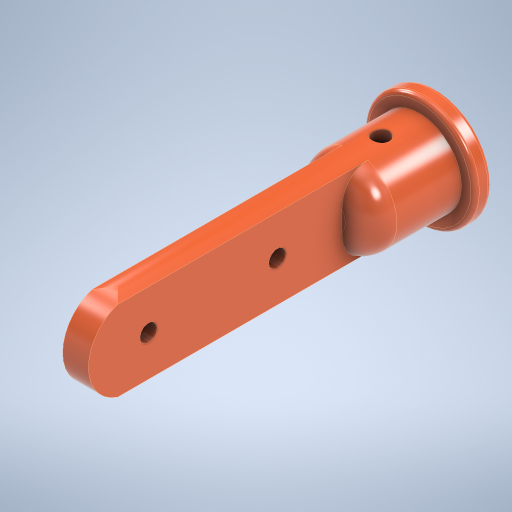
# Autodesk Inventor part: pin
Saved by Autodesk Inventor 2023.2 (Build 272271000, 271)
## iProperties
Created: 2022-11-27
Part Number: pin
Material: Generic
Document SubType Name: Modeling
Designer: omrfrkmll
Density: 1 g/cm^3
Appearance: Smooth - Light Orange
Author: omrfrkmll
Autodesk Inventor part; units mm, degrees
ref_plane "YZ Plane" through (0, 0, 0) normal (1, 0, 0) x (0, 1, 0)
ref_plane "XZ Plane" through (0, 0, 0) normal (0, 1, 0) x (-1, 0, 0)
ref_plane "XY Plane" through (0, 0, 0) normal (0, 0, 1) x (1, 0, 0)
sketch "Sketch2" plane through (0, 0, 0) normal (0, 0, 1) x (1, 0, 0)
  circle A0 centre (0, 0) radius 6.5
  dimension "d0" = 13
  constraints: 1 centre point, 1 coincident
  measures "d0" diameter of A0
extrude "Extrusion1" add sketch "Sketch2" along normal blind 2
sketch "Sketch3" plane through (0, 0, 2) normal (0, 0, 1) x (1, 0, 0)
  circle A0 centre (0, 0) radius 4.9
  dimension "d3" = 9.8
  constraints: 1 centre point, 1 coincident
  measures "d3" diameter of A0
extrude "Extrusion2" add sketch "Sketch3" along normal blind 40
sketch "Sketch4" plane through (0, 0, 0) normal (0, 1, 0) x (-1, 0, 0)
  circle A0 centre (0, 6.5) radius 1
  line L0 (-7.9245, 0) -> (9.7387, 0)
  point P0 (0, 0)
  dimension "d6" = 13
  dimension "d7" = 2
  constraints: 2 end point, 2 horizontal, 1 centre point
  measures "d6" diameter of A0.centre L0
  measures "d7" diameter of A0
extrude "Extrusion3" cut sketch "Sketch4" along normal through all both and the other way through all
fillet "Fillet1" radius 0.5 2 edges at (-6.5, 0, 2) (-6.5, 0, 0)
sketch "Sketch6" plane through (0, 0, 0) normal (0, 1, 0) x (-1, 0, 0)
  line L0 (0, -9.5218) -> (0, 46.9699)
  line L1 (-1.5, 47.9812) -> (-7.2038, 47.9812)
  line L2 (-7.2038, 47.9812) -> (-7.2038, 12.5)
  line L3 (-7.2038, 12.5) -> (-1.5, 12.5)
  line L4 (-1.5, 12.5) -> (-1.5, 47.9812)
  line L5 (1.5, 47.9812) -> (7.2038, 47.9812)
  line L6 (7.2038, 47.9812) -> (7.2038, 12.5)
  line L7 (7.2038, 12.5) -> (1.5, 12.5)
  line L8 (1.5, 12.5) -> (1.5, 47.9812)
  line L9 (-10.513, 0) -> (10.0442, 0)
  point P0 (0, 0)
  dimension "d11" = 3
  dimension "d12" = 0
  dimension "d13" = 25
  constraints: 20 end point, 4 horizontal, 4 parallel, 2 equal length, 2 perpendicular, 2 vertical, 1 other
  measures "d11" distance between parallel lines of L8 L4
  measures "d12" distance between parallel lines of L3 L7
  measures "d13" diameter of L3 L9
extrude "Extrusion4" cut sketch "Sketch6" along normal through all both and the other way through all
sketch "Sketch8" plane through (0, 0, 0) normal (1, 0, 0) x (0, 1, 0)
  line L0 (0, -5.8529) -> (0, 47.5717)
  line L1 (12.046, 0) -> (-11.978, 0)
  circle A0 centre (0, 20) radius 1
  circle A1 centre (0, 35) radius 1
  point P0 (0, 0)
  dimension "d16" = 15
  dimension "d17" = 40
  dimension "d20" = 2
  constraints: 4 end point, 2 centre point, 2 horizontal, 2 point on line, 2 vertical, 1 equal radius
  measures "d16" distance of A0.centre A1.centre
  measures "d17" diameter of A0.centre L1
  measures "d20" diameter of A0
extrude "Extrusion5" cut sketch "Sketch8" along normal mid plane 10
fillet "Fillet2" radius 3 3 edges at (3.9598, -2.8862, 12.5) (3.9598, 2.8862, 12.5) (-4.9, 0, 12.5)
sketch "Sketch9" plane through (1.5, -4.6648, 42) normal (1, 0, 0) x (0, 0, -1)
  circle A0 centre (4.9, 4.6648) radius 4.9
  line L0 (40, 9.5648) -> (0, 9.5648) projected
  line L1 (0, 0) -> (0, 9.3295) projected
  line L2 (4.9, 9.5648) -> (0, 9.5648)
  line L3 (0, 9.5648) -> (0, -0.2352)
  line L4 (0, -0.2352) -> (4.9, -0.2352)
  line L5 (40, -0.2352) -> (0, -0.2352) projected
  point P0 (42, 4.6648)
  point P1 (0, 4.6648)
  constraints: 6 end point, 3 tangent, 2 point on circle, 2 point on line, 1 centre point, 1 collinear, 1 vertical
extrude "Extrusion6" cut sketch "Sketch9" against normal blind 10 contours A0 L1 L3 L0 | L4 L3 L1 A0
body "Solid1"
